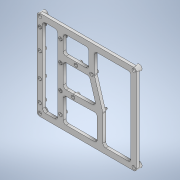
# Autodesk Inventor part: ElectronicsPlate
Saved by Autodesk Inventor 2021 (Build 250183000, 183)
## iProperties
Created: 2021-01-04
Part Number: ElectronicsPlate
Material: Generic
Document SubType Name: Modeling
Designer: elmar
Density: 1 g/cm^3
Appearance: Default
Author: elmar
Autodesk Inventor part; units mm, degrees
ref_plane "YZ Plane" through (0, 0, 0) normal (1, 0, 0) x (0, 1, 0)
ref_plane "XZ Plane" through (0, 0, 0) normal (0, 1, 0) x (-1, 0, 0)
ref_plane "XY Plane" through (0, 0, 0) normal (0, 0, 1) x (1, 0, 0)
sketch "Sketch1" plane through (0, 0, 0) normal (0, 0, 1) x (1, 0, 0)
  spline S0 degree 3 poles (112.5987, 40.5716) (112.8804, 40.5635) (113.1578, 40.5212) (113.7048, 40.3714) (113.9183, 40.2798) (114.0681, 40.2161) knots 0 0 0 0 0.501408 0.501408 1 1 1 1
  spline S1 degree 3 poles (114.0681, 40.2161) (114.4496, 40.0537) (114.795, 39.8169) (115.3917, 39.2131) (115.6321, 38.8467) (115.9696, 38.026) (116.0568, 37.5767) (116.0578, 36.6507) (115.9642, 36.1828) (115.6521, 35.4199) (115.4735, 35.1152) (115.0319, 34.5559) (114.769, 34.3056) (114.4755, 34.0949) knots 0 0 0 0 0.124388 0.124388 0.254428 0.254428 0.390118 0.390118 0.531456 0.531456 0.636484 0.636484 0.744398 0.744398 0.744398 0.744398
  spline S2 degree 3 poles (114.4755, 34.0949) (114.3199, 33.9832) (114.0605, 33.829) (113.3259, 33.5701) (112.9187, 33.5013) (112.5105, 33.5002) knots 0 0 0 0 0.477772 0.477772 1 1 1 1
  spline S3 degree 3 poles (112.5105, 33.5002) (112.1023, 33.4991) (111.6948, 33.5658) (110.9589, 33.8208) (110.6987, 33.9737) (110.5424, 34.0846) knots 0 0 0 0 0.522152 0.522152 1 1 1 1
  spline S4 degree 3 poles (110.5424, 34.0846) (110.1339, 34.3746) (109.7848, 34.7402) (109.2598, 35.5705) (109.0828, 36.0231) (108.9191, 36.9525) (108.9268, 37.4191) (109.1202, 38.3034) (109.2968, 38.7141) (109.722, 39.3292) (109.9292, 39.5551) (110.3934, 39.9358) (110.6465, 40.0908) (110.9177, 40.2078) knots 0 0 0 0 0.150301 0.150301 0.294935 0.294935 0.433898 0.433898 0.567191 0.567191 0.659024 0.659024 0.747992 0.747992 0.747992 0.747992
  spline S5 degree 3 poles (110.9177, 40.2078) (111.0671, 40.2723) (111.28, 40.365) (111.8263, 40.5177) (112.1035, 40.5615) (112.3852, 40.571) knots 0 0 0 0 0.49851 0.49851 1 1 1 1
  arc A0 (112.5987, 40.5716) -> (112.3852, 40.571) centre (112.5, 37.5) ccw
  spline S6 degree 3 poles (37.5987, 115.5716) (37.8804, 115.5635) (38.1578, 115.5212) (38.7048, 115.3714) (38.9183, 115.2798) (39.0681, 115.2161) knots 0 0 0 0 0.501408 0.501408 1 1 1 1
  spline S7 degree 3 poles (39.0681, 115.2161) (39.4496, 115.0537) (39.795, 114.8169) (40.3917, 114.2131) (40.6321, 113.8467) (40.9696, 113.026) (41.0568, 112.5767) (41.0578, 111.6507) (40.9642, 111.1828) (40.6521, 110.4199) (40.4735, 110.1152) (40.0319, 109.5559) (39.769, 109.3056) (39.4755, 109.0949) knots 0 0 0 0 0.124388 0.124388 0.254428 0.254428 0.390118 0.390118 0.531456 0.531456 0.636484 0.636484 0.744398 0.744398 0.744398 0.744398
  spline S8 degree 3 poles (39.4755, 109.0949) (39.3199, 108.9832) (39.0605, 108.829) (38.3259, 108.5701) (37.9187, 108.5013) (37.5105, 108.5002) knots 0 0 0 0 0.477772 0.477772 1 1 1 1
  spline S9 degree 3 poles (37.5105, 108.5002) (37.1023, 108.4991) (36.6948, 108.5658) (35.9589, 108.8208) (35.6987, 108.9737) (35.5424, 109.0846) knots 0 0 0 0 0.522152 0.522152 1 1 1 1
  spline S10 degree 3 poles (35.5424, 109.0846) (35.1339, 109.3746) (34.7848, 109.7402) (34.2598, 110.5705) (34.0828, 111.0231) (33.9191, 111.9525) (33.9268, 112.4191) (34.1202, 113.3034) (34.2968, 113.7141) (34.722, 114.3292) (34.9292, 114.5551) (35.3934, 114.9358) (35.6465, 115.0908) (35.9177, 115.2078) knots 0 0 0 0 0.150301 0.150301 0.294935 0.294935 0.433898 0.433898 0.567191 0.567191 0.659024 0.659024 0.747992 0.747992 0.747992 0.747992
  spline S11 degree 3 poles (35.9177, 115.2078) (36.0671, 115.2723) (36.28, 115.365) (36.8263, 115.5177) (37.1035, 115.5615) (37.3852, 115.571) knots 0 0 0 0 0.49851 0.49851 1 1 1 1
  arc A1 (37.5987, 115.5716) -> (37.3852, 115.571) centre (37.5, 112.5) ccw
  spline S12 degree 3 poles (112.5987, 115.5716) (112.8804, 115.5635) (113.1578, 115.5212) (113.7048, 115.3714) (113.9183, 115.2798) (114.0681, 115.2161) knots 0 0 0 0 0.501408 0.501408 1 1 1 1
  spline S13 degree 3 poles (114.0681, 115.2161) (114.4496, 115.0537) (114.795, 114.8169) (115.3917, 114.2131) (115.6321, 113.8467) (115.9696, 113.026) (116.0568, 112.5767) (116.0578, 111.6507) (115.9642, 111.1828) (115.6521, 110.4199) (115.4735, 110.1152) (115.0319, 109.5559) (114.769, 109.3056) (114.4755, 109.0949) knots 0 0 0 0 0.124388 0.124388 0.254428 0.254428 0.390118 0.390118 0.531456 0.531456 0.636484 0.636484 0.744398 0.744398 0.744398 0.744398
  spline S14 degree 3 poles (114.4755, 109.0949) (114.3199, 108.9832) (114.0605, 108.829) (113.3259, 108.5701) (112.9187, 108.5013) (112.5105, 108.5002) knots 0 0 0 0 0.477772 0.477772 1 1 1 1
  spline S15 degree 3 poles (112.5105, 108.5002) (112.1023, 108.4991) (111.6948, 108.5658) (110.9589, 108.8208) (110.6987, 108.9737) (110.5424, 109.0846) knots 0 0 0 0 0.522152 0.522152 1 1 1 1
  spline S16 degree 3 poles (110.5424, 109.0846) (110.1339, 109.3746) (109.7848, 109.7402) (109.2598, 110.5705) (109.0828, 111.0231) (108.9191, 111.9525) (108.9268, 112.4191) (109.1202, 113.3034) (109.2968, 113.7141) (109.722, 114.3292) (109.9292, 114.5551) (110.3934, 114.9358) (110.6465, 115.0908) (110.9177, 115.2078) knots 0 0 0 0 0.150301 0.150301 0.294935 0.294935 0.433898 0.433898 0.567191 0.567191 0.659024 0.659024 0.747992 0.747992 0.747992 0.747992
  spline S17 degree 3 poles (110.9177, 115.2078) (111.0671, 115.2723) (111.28, 115.365) (111.8263, 115.5177) (112.1035, 115.5615) (112.3852, 115.571) knots 0 0 0 0 0.49851 0.49851 1 1 1 1
  arc A2 (112.5987, 115.5716) -> (112.3852, 115.571) centre (112.5, 112.5) ccw
  spline S18 degree 3 poles (75.0987, 78.0716) (75.3804, 78.0635) (75.6578, 78.0212) (76.2048, 77.8714) (76.4183, 77.7798) (76.5681, 77.7161) knots 0 0 0 0 0.501408 0.501408 1 1 1 1
  spline S19 degree 3 poles (76.5681, 77.7161) (76.9496, 77.5537) (77.295, 77.3169) (77.8917, 76.7131) (78.1321, 76.3467) (78.4696, 75.526) (78.5568, 75.0767) (78.5578, 74.1507) (78.4642, 73.6828) (78.1521, 72.9199) (77.9735, 72.6152) (77.5319, 72.0559) (77.269, 71.8056) (76.9755, 71.5949) knots 0 0 0 0 0.124388 0.124388 0.254428 0.254428 0.390118 0.390118 0.531456 0.531456 0.636484 0.636484 0.744398 0.744398 0.744398 0.744398
  spline S20 degree 3 poles (76.9755, 71.5949) (76.8199, 71.4832) (76.5605, 71.329) (75.8259, 71.0701) (75.4187, 71.0013) (75.0105, 71.0002) knots 0 0 0 0 0.477772 0.477772 1 1 1 1
  spline S21 degree 3 poles (75.0105, 71.0002) (74.6023, 70.9991) (74.1948, 71.0658) (73.4589, 71.3208) (73.1987, 71.4737) (73.0424, 71.5846) knots 0 0 0 0 0.522152 0.522152 1 1 1 1
  spline S22 degree 3 poles (73.0424, 71.5846) (72.6339, 71.8746) (72.2848, 72.2402) (71.7598, 73.0705) (71.5828, 73.5231) (71.4191, 74.4525) (71.4268, 74.9191) (71.6202, 75.8034) (71.7968, 76.2141) (72.222, 76.8292) (72.4292, 77.0551) (72.8934, 77.4358) (73.1465, 77.5908) (73.4177, 77.7078) knots 0 0 0 0 0.150301 0.150301 0.294935 0.294935 0.433898 0.433898 0.567191 0.567191 0.659024 0.659024 0.747992 0.747992 0.747992 0.747992
  spline S23 degree 3 poles (73.4177, 77.7078) (73.5671, 77.7723) (73.78, 77.865) (74.3263, 78.0177) (74.6035, 78.0615) (74.8852, 78.071) knots 0 0 0 0 0.49851 0.49851 1 1 1 1
  arc A3 (75.0987, 78.0716) -> (74.8852, 78.071) centre (75, 75) ccw
  spline S24 degree 3 poles (37.5987, 40.5716) (37.8804, 40.5635) (38.1578, 40.5212) (38.7048, 40.3714) (38.9183, 40.2798) (39.0681, 40.2161) knots 0 0 0 0 0.501408 0.501408 1 1 1 1
  spline S25 degree 3 poles (39.0681, 40.2161) (39.4496, 40.0537) (39.795, 39.8169) (40.3917, 39.2131) (40.6321, 38.8467) (40.9696, 38.026) (41.0568, 37.5767) (41.0578, 36.6507) (40.9642, 36.1828) (40.6521, 35.4199) (40.4735, 35.1152) (40.0319, 34.5559) (39.769, 34.3056) (39.4755, 34.0949) knots 0 0 0 0 0.124388 0.124388 0.254428 0.254428 0.390118 0.390118 0.531456 0.531456 0.636484 0.636484 0.744398 0.744398 0.744398 0.744398
  spline S26 degree 3 poles (39.4755, 34.0949) (39.3199, 33.9832) (39.0605, 33.829) (38.3259, 33.5701) (37.9187, 33.5013) (37.5105, 33.5002) knots 0 0 0 0 0.477772 0.477772 1 1 1 1
  spline S27 degree 3 poles (37.5105, 33.5002) (37.1023, 33.4991) (36.6948, 33.5658) (35.9589, 33.8208) (35.6987, 33.9737) (35.5424, 34.0846) knots 0 0 0 0 0.522152 0.522152 1 1 1 1
  spline S28 degree 3 poles (35.5424, 34.0846) (35.1339, 34.3746) (34.7848, 34.7402) (34.2598, 35.5705) (34.0828, 36.0231) (33.9191, 36.9525) (33.9268, 37.4191) (34.1202, 38.3034) (34.2968, 38.7141) (34.722, 39.3292) (34.9292, 39.5551) (35.3934, 39.9358) (35.6465, 40.0908) (35.9177, 40.2078) knots 0 0 0 0 0.150301 0.150301 0.294935 0.294935 0.433898 0.433898 0.567191 0.567191 0.659024 0.659024 0.747992 0.747992 0.747992 0.747992
  spline S29 degree 3 poles (35.9177, 40.2078) (36.0671, 40.2723) (36.28, 40.365) (36.8263, 40.5177) (37.1035, 40.5615) (37.3852, 40.571) knots 0 0 0 0 0.49851 0.49851 1 1 1 1
  arc A4 (37.5987, 40.5716) -> (37.3852, 40.571) centre (37.5, 37.5) ccw
  circle A5 centre (0, 0) radius 1.6
  circle A6 centre (167.9325, 150) radius 1.6
  circle A7 centre (0, 150) radius 1.6
  circle A8 centre (167.9325, 0) radius 1.6
  circle A9 centre (151.7825, 90.5482) radius 11.5
  circle A10 centre (75, 0) radius 3.15
  circle A11 centre (75, 150) radius 3.15
  circle A12 centre (150, 75) radius 3.15
  circle A13 centre (0, 75) radius 3.15
  circle A14 centre (136.2825, 75.0482) radius 1.6
  circle A15 centre (167.2825, 106.0482) radius 1.6
  circle A16 centre (136.2825, 106.0482) radius 1.6
  circle A17 centre (167.2825, 75.0482) radius 1.6
  arc A18 (-5, 0) -> (0, -5) centre (0, 0) ccw
  line L0 (0, -5) -> (167.9325, -5)
  arc A19 (167.9325, -5) -> (172.9325, 0) centre (167.9325, 0) ccw
  line L1 (172.9325, 0) -> (172.9325, 150)
  arc A20 (172.9325, 150) -> (167.9325, 155) centre (167.9325, 150) ccw
  line L2 (167.9325, 155) -> (0, 155)
  arc A21 (0, 155) -> (-5, 150) centre (0, 150) ccw
  line L3 (-5, 150) -> (-5, 0)
extrude "Extrusion1" add sketch "Sketch1" along normal blind 5 contours S0 S1 S2 S3 S4 S5 A0 | S6 S7 S8 S9 S10 S11 A1 | S12 S13 S14 S15 S16 S17 A2 | S18 S19 S20 S21 S22 S23 A3 | S24 S25 S26 S27 S28 S29 A4 | A5 | A6 | A7 | A8 | A9 | A10 | A11 | A12 | A13 | A14 | A15 | A16 | A17 | L3 A21 L2 A20 L1 A19 L0 A18
sketch "Sketch2" plane through (0, 0, 5) normal (0, 0, 1) x (1, 0, 0)
  arc A0 (0, 155) -> (-5, 150) centre (0, 150) ccw projected
  arc A1 (172.9325, 150) -> (167.9325, 155) centre (167.9325, 150) ccw projected
  arc A2 (167.9325, -5) -> (172.9325, 0) centre (167.9325, 0) ccw projected
  arc A3 (-5, 0) -> (0, -5) centre (0, 0) ccw projected
hole "Hole1" at (0, 150, 5) at (0, 0, 5) at (167.9325, 0, 5) at (167.9325, 150, 5) direction (0, 0, -1) diameter 3.4036 end through all countersink diameter 6.35 countersink angle 90 clearance for "Flat Head Machine Screw" size "M3" standard "Ansi Metric M Profile"
sketch "Sketch3" plane through (0, 0, 0) normal (0, 0, 1) x (1, 0, 0)
  line L0 (37, 96.5) -> (0, 96.5)
  line L1 (0, 96.5) -> (0, 133.5)
  line L2 (0, 133.5) -> (37, 133.5)
  line L3 (37, 133.5) -> (37, 96.5)
  line L4 (37, 96.5) -> (0, 133.5) construction
  line L5 (0, 96.5) -> (37, 133.5) construction
  line L6 (37, 16.5) -> (0, 16.5)
  line L7 (0, 16.5) -> (0, 53.5)
  line L8 (0, 53.5) -> (37, 53.5)
  line L9 (37, 53.5) -> (37, 16.5)
  line L10 (37, 16.5) -> (0, 53.5) construction
  line L11 (0, 16.5) -> (37, 53.5) construction
  line L12 (167.9325, 155) -> (0, 155) projected
  line L13 (0, -5) -> (167.9325, -5) projected
  line L14 (-5, 150) -> (-5, 0) projected
  line L15 (110, 109.29) -> (57, 109.29)
  line L16 (57, 109.29) -> (57, 40.71)
  line L17 (57, 40.71) -> (110, 40.71)
  line L18 (110, 40.71) -> (110, 109.29)
  line L19 (110, 109.29) -> (57, 40.71) construction
  line L20 (57, 109.29) -> (110, 40.71) construction
  line L21 (-5, 150) -> (-5, 0) projected
  line L22 (0, -5) -> (167.9325, -5) projected
  circle A0 centre (0, 16.5) radius 2.75
  circle A1 centre (37, 16.5) radius 2.75
  circle A2 centre (37, 53.5) radius 2.75
  circle A3 centre (0, 53.5) radius 2.75
  circle A4 centre (37, 96.5) radius 2.75
  circle A5 centre (0, 96.5) radius 2.75
  circle A6 centre (0, 133.5) radius 2.75
  circle A7 centre (37, 133.5) radius 2.75
  circle A8 centre (107.8, 55.95) radius 2.25
  circle A9 centre (59.54, 54.68) radius 2.75
  circle A10 centre (92.56, 106.75) radius 2.75
  circle A11 centre (64.62, 106.75) radius 2.75
  point P0 (0, 0)
  point P1 (18.5, 115)
  point P2 (18.5, 35)
  point P3 (83.5, 75)
  point P4 (110, 56.4217)
  point P5 (110, 55.4783)
  point P6 (63.566, 109.29)
  point P7 (65.674, 109.29)
  point P8 (91.506, 109.29)
  point P9 (93.614, 109.29)
  dimension "d9" = 37
  dimension "d10" = 40
  dimension "d11" = 40
  dimension "d13" = 68.58
  dimension "d14" = 53
  dimension "d15" = 5
  dimension "d16" = 20
  dimension "d17" = 80
  dimension "d20" = 66.04
  dimension "d21" = 66.04
  dimension "d23" = 13.97
  dimension "d25" = 15.24
  dimension "d27" = 7.62
  dimension "d28" = 35.56
  dimension "d29" = 2.54
  dimension "d30" = 50.8
  dimension "d31" = 5.5
  dimension "d32" = 4.5
  constraints: 36 end point, 12 centre point, 12 coincident, 10 equal radius, 6 midpoint, 6 parallel, 3 equal length, 3 horizontal, 3 perpendicular, 1 collinear
  measures "d9" distance of L1.end L2.end
  measures "d10" distance from line of point (18.5, 115) L12
  measures "d11" distance from line of L13 point (18.5, 35)
  measures "d13" distance of L15.end L16.end
  measures "d14" distance of L16.end L17.end
  measures "d15" distance between parallel lines of L1 L21
  measures "d16" distance between parallel lines of L3 L16
  measures "d17" distance from line of point (83.5, 75) L22
  measures "d20" distance from line of point (92.56, 106.75) L17
  measures "d21" distance from line of point (64.62, 106.75) L17
  measures "d23" distance from line of point (59.54, 54.68) L17
  measures "d25" distance from line of L17 point (107.8, 55.95)
  measures "d27" distance from line of point (64.62, 106.75) L16
  measures "d28" distance from line of A10.centre L16
  measures "d29" distance from line of A9.centre L16
  measures "d30" distance from line of point (107.8, 55.95) L16
  measures "d31" diameter of A0
  measures "d32" diameter of A8
extrude "Extrusion2" add sketch "Sketch3" against normal blind 5 contours A5 L1 L0 | L0 L1 A5 | A4 L3 L0 | L0 L3 A4 | A6 L2 L1 | L1 L2 A6 | A7 L2 L3 | L3 L2 A7 | A0 L7 L6 | L6 L7 A0 | A1 L9 L6 | L6 L9 A1 | A3 L8 L7 | L7 L8 A3 | A2 L8 L9 | L9 L8 A2 | A10 L15 | L15 A10 | A8 L18 | L18 A8 | A11 L15 | L15 A11 | A9 L16 | L16 A9
sketch "Sketch4" plane through (37, 133.5, -5) normal (0, 0, -1) x (-1, 0, 0)
  circle A0 centre (-22.54, -78.82) radius 2.75 projected
  circle A1 centre (-55.56, -26.75) radius 2.75 projected
  circle A2 centre (-27.62, -26.75) radius 2.75 projected
  circle A3 centre (0, -37) radius 2.75 projected
  circle A4 centre (37, -37) radius 2.75 projected
  circle A5 centre (0, -80) radius 2.75 projected
  circle A6 centre (37, -80) radius 2.75 projected
  circle A7 centre (37, -117) radius 2.75 projected
  circle A8 centre (0, -117) radius 2.75 projected
  circle A9 centre (0, 0) radius 2.75 projected
  circle A10 centre (37, 0) radius 2.75 projected
  point P0 (37, -133.5)
  point P1 (-56.614, -24.21)
  point P2 (-54.506, -24.21)
  point P3 (-28.674, -24.21)
  point P4 (-26.566, -24.21)
hole "Hole2" at (92.56, 106.75, -5) at (64.62, 106.75, -5) at (37, 133.5, -5) at (0, 133.5, -5) at (37, 96.5, -5) at (0, 96.5, -5) at (59.54, 54.68, -5) at (37, 53.5, -5) at (0, 53.5, -5) at (0, 16.5, -5) at (37, 16.5, -5) direction (0, 0, 1) diameter 3.2 end through all
sketch "Sketch5" plane through (0, 0, -5) normal (0, 0, -1) x (-1, 0, 0)
  circle A0 centre (-107.8, 55.95) radius 2.25 projected
  circle A1 centre (-107.8, 55.95) radius 1.55
  point P0 (0, 0)
  point P1 (-110, 55.4783)
  point P2 (-110, 56.4217)
  dimension "d42" = 3.1
  constraints: 1 centre point, 1 coincident
  measures "d42" diameter of A1
extrude "Extrusion3" add sketch "Sketch5" along normal blind 1.5875 contours A1
sketch "Sketch6" plane through (0, 0, 5) normal (0, 0, 1) x (1, 0, 0)
  circle A0 centre (0, 16.5) radius 1.6 projected
  circle A1 centre (37, 16.5) radius 1.6 projected
  circle A2 centre (37, 53.5) radius 1.6 projected
  circle A3 centre (0, 53.5) radius 1.6 projected
  circle A4 centre (59.54, 54.68) radius 1.6 projected
  circle A5 centre (64.62, 106.75) radius 1.6 projected
  circle A6 centre (92.56, 106.75) radius 1.6 projected
  circle A7 centre (37, 96.5) radius 1.6 projected
  circle A8 centre (0, 96.5) radius 1.6 projected
  circle A9 centre (0, 133.5) radius 1.6 projected
  circle A10 centre (0, 133.5) radius 1.6 projected
  line L0 (2.8, 135.1166) -> (2.8, 131.8834)
  line L1 (2.8, 131.8834) -> (0, 130.2668)
  line L2 (0, 130.2668) -> (-2.8, 131.8834)
  line L3 (-2.8, 131.8834) -> (-2.8, 135.1166)
  line L4 (-2.8, 135.1166) -> (0, 136.7332)
  line L5 (0, 136.7332) -> (2.8, 135.1166)
  circle A11 centre (0, 96.5) radius 2.75 projected
  line L6 (2.8, 98.1166) -> (2.8, 94.8834)
  line L7 (2.8, 94.8834) -> (0, 93.2668)
  line L8 (0, 93.2668) -> (-2.8, 94.8834)
  line L9 (-2.8, 94.8834) -> (-2.8, 98.1166)
  line L10 (-2.8, 98.1166) -> (0, 99.7332)
  line L11 (0, 99.7332) -> (2.8, 98.1166)
  line L12 (34.2, 98.1166) -> (37, 99.7332)
  line L13 (37, 99.7332) -> (39.8, 98.1166)
  line L14 (39.8, 98.1166) -> (39.8, 94.8834)
  line L15 (39.8, 94.8834) -> (37, 93.2668)
  line L16 (37, 93.2668) -> (34.2, 94.8834)
  line L17 (34.2, 94.8834) -> (34.2, 98.1166)
  line L18 (61.82, 108.3666) -> (64.62, 109.9832)
  line L19 (64.62, 109.9832) -> (67.42, 108.3666)
  line L20 (67.42, 108.3666) -> (67.42, 105.1334)
  line L21 (67.42, 105.1334) -> (64.62, 103.5168)
  line L22 (64.62, 103.5168) -> (61.82, 105.1334)
  line L23 (61.82, 105.1334) -> (61.82, 108.3666)
  line L24 (92.56, 109.9832) -> (95.36, 108.3666)
  line L25 (95.36, 108.3666) -> (95.36, 105.1334)
  line L26 (95.36, 105.1334) -> (92.56, 103.5168)
  line L27 (92.56, 103.5168) -> (89.76, 105.1334)
  line L28 (89.76, 105.1334) -> (89.76, 108.3666)
  line L29 (89.76, 108.3666) -> (92.56, 109.9832)
  line L30 (59.54, 57.9132) -> (62.34, 56.2966)
  line L31 (62.34, 56.2966) -> (62.34, 53.0634)
  line L32 (62.34, 53.0634) -> (59.54, 51.4468)
  line L33 (59.54, 51.4468) -> (56.74, 53.0634)
  line L34 (56.74, 53.0634) -> (56.74, 56.2966)
  line L35 (56.74, 56.2966) -> (59.54, 57.9132)
  circle A12 centre (37, 53.5) radius 1.6 projected
  line L36 (34.2, 55.1166) -> (37, 56.7332)
  line L37 (37, 56.7332) -> (39.8, 55.1166)
  line L38 (39.8, 55.1166) -> (39.8, 51.8834)
  line L39 (39.8, 51.8834) -> (37, 50.2668)
  line L40 (37, 50.2668) -> (34.2, 51.8834)
  line L41 (34.2, 51.8834) -> (34.2, 55.1166)
  circle A13 centre (0, 53.5) radius 1.6 projected
  line L42 (0, 56.7332) -> (2.8, 55.1166)
  line L43 (2.8, 55.1166) -> (2.8, 51.8834)
  line L44 (2.8, 51.8834) -> (0, 50.2668)
  line L45 (0, 50.2668) -> (-2.8, 51.8834)
  line L46 (-2.8, 51.8834) -> (-2.8, 55.1166)
  line L47 (-2.8, 55.1166) -> (0, 56.7332)
  line L48 (2.8, 18.1166) -> (2.8, 14.8834)
  line L49 (2.8, 14.8834) -> (0, 13.2668)
  line L50 (0, 13.2668) -> (-2.8, 14.8834)
  line L51 (-2.8, 14.8834) -> (-2.8, 18.1166)
  line L52 (-2.8, 18.1166) -> (0, 19.7332)
  line L53 (0, 19.7332) -> (2.8, 18.1166)
  line L54 (34.2, 14.8834) -> (34.2, 18.1166)
  line L55 (34.2, 18.1166) -> (37, 19.7332)
  line L56 (37, 19.7332) -> (39.8, 18.1166)
  line L57 (39.8, 18.1166) -> (39.8, 14.8834)
  line L58 (39.8, 14.8834) -> (37, 13.2668)
  line L59 (37, 13.2668) -> (34.2, 14.8834)
  circle A14 centre (37, 133.5) radius 1.6 projected
  circle A15 centre (37, 133.5) radius 1.6 projected
  line L60 (34.2, 135.1166) -> (37, 136.7332)
  line L61 (37, 136.7332) -> (39.8, 135.1166)
  line L62 (39.8, 135.1166) -> (39.8, 131.8834)
  line L63 (39.8, 131.8834) -> (37, 130.2668)
  line L64 (37, 130.2668) -> (34.2, 131.8834)
  line L65 (34.2, 131.8834) -> (34.2, 135.1166)
  point P0 (0, 0)
  dimension "d45" = 5.6
  constraints: 132 end point, 11 coincident, 11 vertical, 10 equal length, 143 other
  measures "d45" distance between parallel lines of L62 L65
extrude "Extrusion4" cut sketch "Sketch6" against normal blind 4 contours A0 | A1 | A2 | A3 | A4 | A5 | A6 | A7 | A8 | A9 | L0 L1 L2 L3 L4 L5 | A11 | L6 L7 L8 L9 L10 L11 | L12 L13 L14 L15 L16 L17 | L18 L19 L20 L21 L22 L23 | L24 L25 L26 L27 L28 L29 | L30 L31 L32 L33 L34 L35 | L36 L37 L38 L39 L40 L41 | L42 L43 L44 L45 L46 L47 | L48 L49 L50 L51 L52 L53 | L54 L55 L56 L57 L58 L59 | A14 | L60 L61 L62 L63 L64 L65
sketch "Sketch7" plane through (0, 0, 0) normal (0, 0, -1) x (-1, 0, 0)
  circle A0 centre (-167.9325, 150) radius 3.175 projected
  circle A1 centre (0, 150) radius 3.175 projected
  circle A2 centre (-167.9325, 0) radius 3.175 projected
  circle A3 centre (0, 0) radius 3.175 projected
  circle A4 centre (-37, 16.5) radius 2.75 projected
  circle A5 centre (-107.8, 55.95) radius 2.25 projected
  circle A6 centre (-167.9325, 0) radius 1.7018 projected
  circle A7 centre (0, 150) radius 1.7018 projected
  circle A8 centre (0, 0) radius 1.7018 projected
  circle A9 centre (-167.9325, 150) radius 1.7018 projected
  line L0 (0, -5) -> (-167.9325, -5) projected
  arc A10 (0, -5) -> (5, 0) centre (0, 0) ccw projected
  line L1 (5, 150) -> (5, 0) projected
  arc A11 (5, 150) -> (0, 155) centre (0, 150) ccw projected
  line L2 (-167.9325, 155) -> (0, 155) projected
  arc A12 (-167.9325, 155) -> (-172.9325, 150) centre (-167.9325, 150) ccw projected
  line L3 (-172.9325, 0) -> (-172.9325, 150) projected
  arc A13 (-172.9325, 0) -> (-167.9325, -5) centre (-167.9325, 0) ccw projected
  line L4 (-162.9325, 145) -> (-5, 145)
  line L5 (-5, 145) -> (-5, 5)
  line L6 (-5, 5) -> (-162.9325, 5)
  line L7 (-162.9325, 5) -> (-162.9325, 145)
  arc A14 (5, 150) -> (0, 155) centre (0, 150) ccw projected
  line L8 (-32, 5) -> (-42, 5)
  line L9 (-42, 5) -> (-42, 145)
  line L10 (-42, 145) -> (-32, 145)
  line L11 (-32, 145) -> (-32, 5)
  line L12 (-32, 5) -> (-42, 145) construction
  line L13 (-42, 5) -> (-32, 145) construction
  circle A15 centre (-37, 53.5) radius 1.6 projected
  circle A16 centre (-37, 16.5) radius 1.6 projected
  line L14 (-37, 53.5) -> (-37, 16.5)
  line L15 (-87.56, 101.75) -> (-97.56, 101.75)
  line L16 (-97.56, 101.75) -> (-97.56, 145)
  line L17 (-97.56, 145) -> (-87.56, 145)
  line L18 (-87.56, 145) -> (-87.56, 101.75)
  line L19 (-87.56, 101.75) -> (-97.56, 145) construction
  line L20 (-97.56, 101.75) -> (-87.56, 145) construction
  line L21 (-97.56, 101.75) -> (-42, 101.75)
  line L22 (-42, 101.75) -> (-42, 111.75)
  line L23 (-42, 111.75) -> (-97.56, 111.75)
  line L24 (-97.56, 111.75) -> (-97.56, 101.75)
  line L25 (-97.56, 101.75) -> (-42, 111.75) construction
  line L26 (-42, 101.75) -> (-97.56, 111.75) construction
  arc A17 (-91.506, 109.29) -> (-91.506, 109.29) centre (-92.56, 106.75) ccw projected
  line L27 (-92.56, 106.75) -> (-64.62, 106.75)
  line L28 (-64.62, 106.75) -> (-92.56, 106.75)
  circle A18 centre (-92.56, 106.75) radius 1.6 projected
  line L29 (-92.56, 106.75) -> (-92.56, 145)
  line L30 (-42, 49.68) -> (-64.54, 49.68)
  line L31 (-64.54, 49.68) -> (-64.54, 59.68)
  line L32 (-64.54, 59.68) -> (-42, 59.68)
  line L33 (-42, 59.68) -> (-42, 49.68)
  line L34 (-42, 49.68) -> (-64.54, 59.68) construction
  line L35 (-64.54, 49.68) -> (-42, 59.68) construction
  line L36 (-97.56, 107.4838) -> (-87.9817, 104.6104)
  line L37 (-87.9817, 104.6104) -> (-103.0109, 54.5133)
  line L38 (-103.0109, 54.5133) -> (-112.5891, 57.3867)
  line L39 (-112.5891, 57.3867) -> (-97.56, 107.4838)
  line L40 (-107.6685, 60.9483) -> (-107.9315, 50.9517)
  line L41 (-107.9315, 50.9517) -> (-59.6058, 49.68)
  line L42 (-59.6058, 49.68) -> (-59.3427, 59.6765)
  line L43 (-59.3427, 59.6765) -> (-107.6685, 60.9483)
  line L44 (-92.7709, 106.0471) -> (-107.8, 55.95)
  line L45 (-107.8, 55.95) -> (-59.4742, 54.6783)
  circle A19 centre (-59.54, 54.68) radius 1.6 projected
  line L46 (-59.54, 54.68) -> (-42, 54.68)
  circle A20 centre (-107.8, 55.95) radius 5
  line L47 (-102.8, 5) -> (-112.8, 5)
  line L48 (-112.8, 5) -> (-112.8, 55.95)
  line L49 (-112.8, 55.95) -> (-102.8, 55.95)
  line L50 (-102.8, 55.95) -> (-102.8, 5)
  line L51 (-102.8, 5) -> (-112.8, 55.95) construction
  line L52 (-112.8, 5) -> (-102.8, 55.95) construction
  line L53 (-107.8, 30.475) -> (-107.8, 55.95)
  point P0 (-37, 75)
  point P1 (-37, 75)
  point P2 (-92.56, 123.375)
  point P3 (-69.78, 106.75)
  point P4 (-92.56, 123.375)
  point P5 (-69.78, 106.75)
  point P6 (-53.27, 54.68)
  point P7 (-53.27, 54.68)
  point P8 (-102.8, 50.8167)
  point P9 (-64.54, 49.8098)
  point P10 (-87.56, 111.75)
  point P11 (-101.132, 60.7763)
  point P12 (-59.4742, 59.68)
  point P13 (-88.8398, 101.75)
  dimension "d48" = 10
  dimension "d49" = 10
  dimension "d50" = 10
  dimension "d51" = 10
  dimension "d52" = 5
  dimension "d53" = 10
  dimension "d54" = 10
  dimension "d55" = 10
  dimension "d56" = 10
  constraints: 100 end point, 20 midpoint, 15 equal length, 15 point on line, 13 perpendicular, 6 horizontal, 5 collinear, 4 tangent, 3 point on circle, 1 centre point, 1 coincident, 1 vertical
  measures "d48" distance between parallel lines of L11 L9
  measures "d49" distance between parallel lines of L21 L23
  measures "d50" distance of L15.start L15.end
  measures "d51" distance of L32.end L30.start
  measures "d52" distance from line of L31 point (-59.54, 54.68)
  measures "d53" distance of L41.end L42.end
  measures "d54" distance of L37.end L38.end
  measures "d55" diameter of A20
  measures "d56" distance between parallel lines of L50 L48
extrude "Extrusion5" cut sketch "Sketch7" against normal through all contours A20 L48 L6 L7 L4 L16 L39 | L37 L15 L21 L9 L32 L43 | L41 L31 L30 L9 L6 L50 | L11 L4 L5 L6 | L18 L4 L9 L23
fillet "Fillet1" radius 5 22 edges at (5, 5, 2.5) (42, 5, 2.5) (112.8, 5, 2.5) (97.56, 107.4838, 2.5) (42, 111.75, 2.5) (42, 59.68, 2.5) (59.4742, 59.68, 2.5) (162.9325, 145, 2.5) (87.56, 145, 2.5) (88.8398, 101.75, 2.5) (102.8, 50.8167, 2.5) (32, 145, 2.5) (97.56, 145, 2.5) (42, 145, 2.5) (5, 145, 2.5) (42, 101.75, 2.5) (42, 49.68, 2.5) (162.9325, 5, 2.5) (101.132, 60.7763, 2.5) (87.56, 111.75, 2.5) (32, 5, 2.5) (102.8, 5, 2.5)
sketch "Sketch8" plane through (0, 0, 0) normal (0, 0, -1) x (-1, 0, 0)
  circle A0 centre (-167.9325, 150) radius 1.7018 projected
  circle A1 centre (0, 150) radius 1.7018 projected
  circle A2 centre (0, 0) radius 1.7018 projected
  circle A3 centre (-167.9325, 0) radius 1.7018 projected
  circle A4 centre (-167.9325, 150) radius 5
  circle A5 centre (0, 150) radius 5
  circle A6 centre (-167.9325, 0) radius 5
  circle A7 centre (0, 0) radius 5
  line L0 (-167.9325, 155) -> (0, 155) projected
  constraints: 4 centre point, 3 equal radius, 1 tangent
extrude "Extrusion6" add sketch "Sketch8" along normal up to surface (5 mm away)
body "Solid1"
